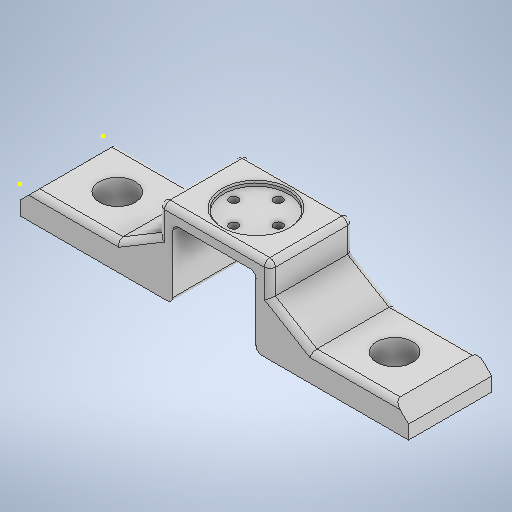
# Autodesk Inventor part: 4_DOF_2
Saved by Autodesk Inventor 2025 (Build 290162000, 162)
## iProperties
Created: 2026-07-06
Part Number: 4_DOF_2
Material: Generic
Document SubType Name: Sheet Metal
Designer: MSI
Density: 1 g/cm^3
Sheet Metal Rule: Default_mm
Appearance: Default
Author: MSI
Autodesk Inventor part; units mm, degrees
ref_plane "YZ Plane" through (0, 0, 0) normal (1, 0, 0) x (0, 1, 0)
ref_plane "XZ Plane" through (0, 0, 0) normal (0, 1, 0) x (-1, 0, 0)
ref_plane "XY Plane" through (0, 0, 0) normal (0, 0, 1) x (1, 0, 0)
sketch "Sketch1" plane through (0, 0, 0) normal (0, 0, 1) x (1, 0, 0)
  line L0 (5, 0) -> (50, 0)
  line L1 (50, 0) -> (50, 18)
  line L2 (52, 20) -> (88, 20)
  line L3 (90, 18) -> (90, 0)
  line L4 (105, 0) -> (135, 0)
  line L5 (140, -5) -> (140, -10)
  line L6 (140, -10) -> (87, -10)
  line L7 (53, -10) -> (0, -10)
  line L8 (0, -10) -> (0, -5)
  line L9 (57, 15) -> (83, 15)
  line L10 (55, 13) -> (55, -8)
  line L11 (85, -8) -> (85, 13)
  arc A0 (52, 20) -> (50, 18) centre (52, 18) ccw
  arc A1 (90, 18) -> (88, 20) centre (88, 18) ccw
  line L12 (50, 9) -> (35, 0)
  line L13 (90, 0) -> (90, 9)
  line L14 (90, 9) -> (105, 0)
  arc A2 (57, 15) -> (55, 13) centre (57, 13) ccw
  arc A3 (85, 13) -> (83, 15) centre (83, 13) ccw
  arc A4 (53, -10) -> (55, -8) centre (53, -8) ccw
  arc A5 (85, -8) -> (87, -10) centre (87, -8) ccw
  line L15 (5, 0) -> (0, -5)
  line L16 (135, 0) -> (140, -5)
  point P0 (0, 0)
  point P1 (50, 20)
  point P2 (90, 20)
  point P3 (140, 0)
  point P4 (140, 0)
  point P5 (0, 0)
  point P6 (140, 0)
  dimension "d0" = 50
  dimension "d1" = 20
  dimension "d2" = 40
  dimension "d3" = 50
  dimension "d4" = 10
  dimension "d7" = 10
  dimension "d8" = 5
  dimension "d9" = 2
  dimension "d10" = 15
  dimension "d11" = 9
  dimension "d12" = 15
  dimension "d13" = 2
  dimension "d14" = 30
  dimension "d15" = 2
  dimension "d18" = 5
  dimension "d19" = 5
  dimension "d20" = 5
  dimension "d21" = 5
  constraints: 34 end point, 17 point on line, 12 point on circle, 12 tangent, 8 perpendicular, 6 centre point, 3 equal radius, 2 midpoint, 1 horizontal, 1 vertical
  measures "d0" distance of point (0, 0) L0.end
  measures "d1" distance of L0.end point (50, 20)
  measures "d2" distance of point (50, 20) point (90, 20)
  measures "d3" distance of L3.end point (140, 0)
  measures "d4" distance of L7.end point (0, 0)
  measures "d7" distance of point (140, 0) L5.end
  measures "d8" distance between parallel lines of L2 L9
  measures "d9" radius of A0
  measures "d10" horizontal distance of L12.start L12.end
  measures "d11" distance of L3.end L13.end
  measures "d12" distance of L4.start L3.end
  measures "d13" radius of A2
  measures "d14" distance of L11.end L10.start
  measures "d15" radius of A4
  measures "d18" distance of L0.start point (0, 0)
  measures "d19" distance of L8.end point (0, 0)
  measures "d20" distance of L4.end point (140, 0)
  measures "d21" distance of L5.start point (140, 0)
extrude "Extrusion1" add sketch "Sketch1" along normal blind 30
sketch "Sketch2" plane through (105, 0, 0) normal (0, 1, 0) x (1, 0, 0)
  circle A0 centre (15, -15) radius 6.5
  line L0 (30, 0) -> (0, 0) projected
  line L1 (0, 0) -> (0, -30) projected
  circle A1 centre (-84.9999, -15) radius 6.5
  line L2 (-100, 0) -> (-100, -30) projected
  line L3 (-70, 0) -> (-100, 0) projected
  point P0 (-105, 0)
  point P1 (0, -15)
  dimension "d24" = 13
  dimension "d25" = 15
  dimension "d26" = 15
  dimension "d27" = 13
  dimension "d28" = 15
  dimension "d29" = 15
  constraints: 2 centre point, 1 midpoint
  measures "d24" diameter of A0
  measures "d25" distance from line of L0 A0.centre
  measures "d26" distance of point (0, -15) A0.centre
  measures "d27" diameter of A1
  measures "d28" distance from line of L2 A1.centre
  measures "d29" distance from line of L3 A1.centre
extrude "Extrusion2" cut sketch "Sketch2" against normal blind 30
sketch "Sketch3" plane through (0, 0, 30) normal (0, 0, 1) x (1, 0, 0)
  point P0 (0, 0)
sketch "Sketch4" plane through (52, 20, 0) normal (0, 1, 0) x (1, 0, 0)
  circle A0 centre (18, -15) radius 11.75
  line L0 (38, 0) -> (38, -30) projected
  line L1 (36, 0) -> (0, 0) projected
  circle A1 centre (18, -7) radius 1.6
  circle A2 centre (10, -15) radius 1.6
  circle A3 centre (18, -23) radius 1.6
  circle A4 centre (26, -15) radius 1.6
  point P0 (-52, 0)
  dimension "d32" = 23.5
  dimension "d33" = 20
  dimension "d34" = 15
  dimension "d35" = 3.2
  dimension "d36" = 8
  dimension "d39" = 360
  constraints: 5 centre point, 2 coincident, 11 other
  measures "d32" diameter of A0
  measures "d33" distance from line of L0 A0.centre
  measures "d34" distance from line of L1 A0.centre
  measures "d35" diameter of A1
  measures "d36" distance of A1.centre A0.centre
extrude "Extrusion3" cut sketch "Sketch4" against normal blind 1.5
extrude "Extrusion4" cut sketch "Sketch4" against normal blind 30 contours A1 | A2 | A3 | A4
fillet "Fillet1" radius 2 18 edges at (50.5858, 19.4142, 0) (50, 13.5, 0) (89.4142, 19.4142, 0) (90, 13.5, 0) (70, 20, 0) (50.5858, 19.4142, 30) (50, 13.5, 30) (89.4142, 19.4142, 30) (90, 13.5, 30) (70, 20, 30) (97.5, 4.5, 30) (120, 0, 30) (97.5, 4.5, 0) (120, 0, 0) (42.5, 4.5, 30) (20, 0, 30) (20, 0, 0) (42.5, 4.5, 0)
chamfer "Chamfer1" distance 0.5 angle 45 1 edges at (58.25, 20, 15)
sketch "Sketch5" plane through (105, 0, 28) normal (0, 1, 0) x (1, 0, 0)
  point P0 (-105, 28)
equation "\"d19\" = d18"
equation "\"d20\" = d18"
equation "\"d21\" = d20"
equation "\"BendRadius\" = Thickness"
equation "\"BendReliefWidth\" = Thickness"
equation "\"BendReliefDepth\" = 0.5 * Thickness"
equation "\"CornerReliefSize\" = 4 * Thickness"
equation "\"MinimumRemnant\" = 2 * Thickness"
equation "\"TransitionRadius\" = BendRadius"
equation "\"JacobiRadiusSize\" = BendRadius"
equation "\"GapSize\" = Thickness"
equation "\"Thickness\" = 0.5"
body "Solid1"
